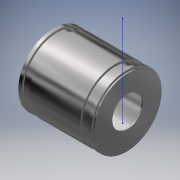
# Autodesk Inventor part: OutsideMiddleShaftCJE
Saved by Autodesk Inventor 2018 (Build 220112000, 112)
## iProperties
Created: 2018-01-21
Part Number: OutsideMiddleShaftCJE
Material: Steel, Alloy
Document SubType Name: Modeling
Designer: textboox5
Density: 7.73 g/cm^3
Appearance: Semi-Polished
Author: textboox5
Autodesk Inventor part; units mm, degrees
ref_plane "YZ Plane" through (0, 0, 0) normal (1, 0, 0) x (0, 1, 0)
ref_plane "XZ Plane" through (0, 0, 0) normal (0, 1, 0) x (-1, 0, 0)
ref_plane "XY Plane" through (0, 0, 0) normal (0, 0, 1) x (1, 0, 0)
sketch "Sketch1" plane through (0, 0, 0) normal (0, 0, 1) x (1, 0, 0)
  line L0 (1524.8384, 1524.0029) -> (1524.8384, 1625.6029)
  line L1 (1524.8384, 1625.6029) -> (1677.2384, 1625.6029)
  line L2 (1677.2384, 1625.6029) -> (1677.2384, 1524.0029)
  line L3 (1677.2384, 1422.4029) -> (-1677.2384, 1422.4029)
  line L4 (-1677.2384, 1524.0029) -> (-1677.2384, 1625.6029)
  line L5 (-1677.2384, 1625.6029) -> (-1524.8384, 1625.6029)
  line L6 (-1524.8384, 1625.6029) -> (-1524.8384, 1524.0029)
  line L7 (0, 0) -> (0, 1422.4029) construction
  line L8 (-1778.8384, 0) -> (1778.8384, 0) construction
  line L9 (-1677.2384, 1524.0029) -> (-1778.8384, 1524.0029)
  line L10 (-1778.8384, 1524.0029) -> (-1778.8384, 711.2)
  line L11 (-1778.8384, 711.2) -> (-1677.2384, 711.2)
  line L12 (-1677.2384, 1422.4029) -> (-1677.2384, 711.2)
  line L13 (1677.2384, 1524.0029) -> (1778.8384, 1524.0029)
  line L14 (1778.8384, 1524.0029) -> (1778.8384, 711.2)
  line L15 (1778.8384, 711.2) -> (1677.2384, 711.2)
  line L16 (1677.2384, 711.2) -> (1677.2384, 1422.4029)
  line L17 (-1169.2384, 1524.0029) -> (-1169.2384, 1625.6029)
  line L18 (-1169.2384, 1625.6029) -> (1169.2384, 1625.6029)
  line L19 (1169.2384, 1625.6029) -> (1169.2384, 1524.0029)
  line L20 (-1524.8384, 1524.0029) -> (-1169.2384, 1524.0029)
  line L21 (1169.2384, 1524.0029) -> (1524.8384, 1524.0029)
  line L22 (0, 711.2) -> (0, -711.2) construction
  line L23 (-1524.8384, -2097.6769) -> (-1524.8384, 2097.6769) construction
  line L24 (1167.5616, -2093.8572) -> (1167.5616, 2101.4966) construction
  line L25 (-1169.2384, 2097.6769) -> (-1169.2384, -2097.6769) construction
  line L26 (1523.1616, 2101.4966) -> (1523.1616, -2093.8572) construction
  line L27 (-1474.0384, -1524.0029) -> (-1474.0384, 1524.0029) construction
  line L28 (-1220.0384, 1524.0029) -> (-1220.0384, -1524.0029) construction
revolve "Revolution1" add sketch "Sketch1" angle 360 about axis through (-1778.8384, 0, 0) along (1, 0, 0)
body "Solid1"
